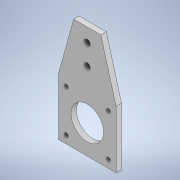
# Autodesk Inventor part: Stepper Motor to Extrusion Clip
Saved by Autodesk Inventor 2022 (Build 260153000, 153)
## iProperties
Created: 2022-12-30
Part Number: Stepper Motor to Extrusion Clip
Material: Generic
Document SubType Name: Modeling
Designer: Gaming
Density: 1 g/cm^3
Appearance: Default
Author: Gaming
Autodesk Inventor part; units mm, degrees
ref_plane "YZ Plane" through (0, 0, 0) normal (1, 0, 0) x (0, 1, 0)
ref_plane "XZ Plane" through (0, 0, 0) normal (0, 1, 0) x (-1, 0, 0)
ref_plane "XY Plane" through (0, 0, 0) normal (0, 0, 1) x (1, 0, 0)
sketch "Sketch1" plane through (0, 0, 0) normal (0, 0, 1) x (1, 0, 0)
  line L0 (21.15, 21.15) -> (21.15, -21.15)
  line L1 (21.15, -21.15) -> (-21.15, -21.15)
  line L2 (-21.15, -21.15) -> (-21.15, 21.15)
  line L3 (-21.15, 21.15) -> (-10, 61.15)
  line L4 (-10, 61.15) -> (10, 61.15)
  line L5 (10, 61.15) -> (21.15, 21.15)
  point P0 (0, 0)
  point P1 (21.15, 0)
  point P2 (0, 61.15)
  dimension "d0" = 42.3
  dimension "d1" = 42.3
  dimension "d2" = 20
  dimension "d4" = 42.3
  dimension "d5" = 40
  dimension "d7" = 11.15
  constraints: 12 end point, 2 midpoint, 2 parallel, 1 equal length, 1 horizontal, 1 horizontal alignment, 1 vertical alignment
  measures "d0" distance of L1.end L2.end
  measures "d1" distance of L0.end L1.end
  measures "d2" distance of L3.end L4.end
  measures "d4" distance of L0.start L2.end
  measures "d5" vertical distance of L3.end L2.end
  measures "d7" horizontal distance of L0.start L4.end
extrude "Extrusion1" add sketch "Sketch1" along normal blind 4
sketch "Sketch2" plane through (0, 0, 4) normal (0, 0, 1) x (1, 0, 0)
  line L0 (10, 61.15) -> (-10, 61.15) projected
  point P0 (0, 0)
  point P1 (0, 51.15)
  point P2 (0, 36.15)
  dimension "d10" = 10
  dimension "d11" = 15
  constraints: 2 vertical alignment
  measures "d10" distance from line of L0 point (0, 51.15)
  measures "d11" distance of point (0, 36.15) point (0, 51.15)
hole "Hole1" at (0, 51.15, 4) at (0, 36.15, 4) direction (0, 0, -1) diameter 4.5 end through all
sketch "Sketch3" plane through (0, 0, 4) normal (0, 0, 1) x (1, 0, 0)
  circle A0 centre (0, 0) radius 12
  dimension "d19" = 24
  constraints: 1 centre point, 1 coincident
  measures "d19" diameter of A0
extrude "Extrusion2" cut sketch "Sketch3" against normal through all
sketch "Sketch4" plane through (0, 0, 4) normal (0, 0, 1) x (1, 0, 0)
  line L0 (-21.15, 21.15) -> (-21.15, -21.15) projected
  line L1 (-21.15, -21.15) -> (21.15, -21.15) projected
  point P0 (0, 0)
  point P1 (-15.5, 15.5)
  point P2 (15.5, 15.5)
  point P3 (15.5, -15.5)
  point P4 (-15.5, -15.5)
  dimension "d22" = 31
  dimension "d23" = 31
  dimension "d24" = 5.65
  dimension "d25" = 5.65
  constraints: 2 horizontal alignment, 2 vertical alignment
  measures "d22" distance of point (15.5, 15.5) point (-15.5, 15.5)
  measures "d23" distance of point (-15.5, -15.5) point (-15.5, 15.5)
  measures "d24" distance from line of L0 point (-15.5, -15.5)
  measures "d25" distance from line of L1 point (-15.5, -15.5)
hole "Hole2" at (-15.5, 15.5, 4) at (15.5, 15.5, 4) at (15.5, -15.5, 4) at (-15.5, -15.5, 4) direction (0, 0, -1) diameter 3 end through all
body "Solid1"
